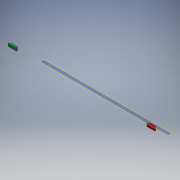
# Autodesk Inventor part: LedCovers
Saved by Autodesk Inventor 2018 (Build 220112000, 112)
## iProperties
Created: 2019-05-03
Part Number: LedCovers
Material: Generic
Document SubType Name: Modeling
Designer: thatg
Density: 1 g/cm^3
Appearance: Default
Author: thatg
Autodesk Inventor part; units mm, degrees
ref_plane "YZ Plane" through (0, 0, 0) normal (1, 0, 0) x (0, 1, 0)
ref_plane "Work Plane1" through (0, 10.16, -2.54) normal (0, -1, 0) x (-1, 0, 0)
ref_plane "Work Plane2" through (-110.49, 8.255, -2.54) normal (0, 1, 0) x (0, 0, 1)
sketch "Sketch2" plane through (0, 10.16, -2.54) normal (0, -1, 0) x (-1, 0, 0)
  line L0 (4.445, -1.27) -> (4.445, -1.905)
  line L1 (3.81, -1.905) -> (4.445, -1.905)
  line L2 (3.81, -2.54) -> (3.81, -1.905)
  line L3 (3.81, -2.54) -> (9.525, -2.54)
  line L4 (9.525, -2.54) -> (9.525, -1.905)
  line L5 (8.89, -1.905) -> (9.525, -1.905)
  line L6 (8.89, -1.27) -> (8.89, -1.905)
  line L7 (8.89, -1.27) -> (4.445, -1.27)
  point P0 (0, -2.54)
extrude "Extrusion1" add sketch "Sketch2" along normal up to surface (1.905 mm away)
sketch "Sketch3" plane through (-4.445, 10.16, -1.27) normal (0, 0, -1) x (-1, 0, 0)
  line L0 (4.445, -1.905) -> (0, -1.905) projected
  line L1 (4.445, 0) -> (4.445, -1.905) projected
  line L2 (4.445, 0) -> (0, 0) projected
  line L3 (0, 0) -> (0, -1.905) projected
  point P0 (-4.445, -10.16)
extrude "Extrusion2" add sketch "Sketch3" along normal blind 0.127
ref_plane "Work Plane3" through (-110.49, 8.255, -2.54) normal (0, 1, 0) x (0, 0, 1)
sketch "Sketch5" plane through (0, 10.16, -2.54) normal (0, -1, 0) x (-1, 0, 0)
  line L0 (100.33, -1.27) -> (100.33, -1.905)
  line L1 (99.695, -1.905) -> (100.33, -1.905)
  line L2 (99.695, -2.54) -> (99.695, -1.905)
  line L3 (99.695, -2.54) -> (105.41, -2.54)
  line L4 (105.41, -2.54) -> (105.41, -1.905)
  line L5 (104.775, -1.905) -> (105.41, -1.905)
  line L6 (104.775, -1.27) -> (104.775, -1.905)
  line L7 (104.775, -1.27) -> (100.33, -1.27)
  point P0 (0, -2.54)
extrude "Extrusion3" add sketch "Sketch5" along normal up to surface (1.905 mm away) separate body
sketch "Sketch6" plane through (-100.33, 10.16, -1.27) normal (0, 0, -1) x (-1, 0, 0)
  line L0 (4.445, -1.905) -> (0, -1.905) projected
  line L1 (4.445, 0) -> (4.445, -1.905) projected
  line L2 (4.445, 0) -> (0, 0) projected
  line L3 (0, 0) -> (0, -1.905) projected
  point P0 (-100.33, -10.16)
extrude "Extrusion4" add sketch "Sketch6" along normal blind 0.127 bodies 2
fillet "Fillet1" radius 0.127 4 edges at (-4.445, 9.2075, -1.397) (-8.89, 9.2075, -1.397) (-6.6675, 8.255, -1.397) (-6.6675, 10.16, -1.397)
fillet "Fillet2" radius 0.127 4 edges at (-100.33, 9.2075, -1.397) (-102.5525, 10.16, -1.397) (-104.775, 9.2075, -1.397) (-102.5525, 8.255, -1.397)
body "Solid1"
body "Solid2"
